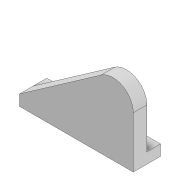
# Autodesk Inventor part: Print_Parts_F1
Saved by Autodesk Inventor 2020 (Build 240168000, 168)
## iProperties
Created: 2020-10-30
Part Number: Print_Parts_F1
Material: Generic
Document SubType Name: Modeling
Designer: magnarecta
Density: 1 g/cm^3
Appearance: Default
Author: magnarecta
Autodesk Inventor part; units mm, degrees
ref_plane "YZ Plane" through (0, 0, 0) normal (1, 0, 0) x (0, 1, 0)
ref_plane "XZ Plane" through (0, 0, 0) normal (0, 1, 0) x (-1, 0, 0)
ref_plane "XY Plane" through (0, 0, 0) normal (0, 0, 1) x (1, 0, 0)
sketch "Sketch1" plane through (0, 0, 0) normal (0, 0, 1) x (1, 0, 0)
  line L0 (0, 0) -> (83.7172, 0)
  line L1 (83.7172, 0) -> (83.7172, 8)
  line L2 (83.7172, 8) -> (0, 8)
  line L3 (0, 8) -> (0, 0)
  line L4 (0, 8) -> (83.7172, 66.6194)
  line L5 (83.7172, 8) -> (83.7172, 66.6194)
  circle A0 centre (68.7172, 37.8047) radius 15
  point P0 (83.7172, 37.8047)
  point P1 (60.1136, 50.092)
  dimension "d0" = 35
  dimension "d1" = 8
  dimension "d12" = 30
  dimension "d13" = 29.8047
  constraints: 12 end point, 2 parallel, 2 tangent, 1 centre point, 1 collinear, 1 horizontal, 1 perpendicular
  measures "d0" angle of L4 L0
  measures "d1" distance of L0.end L1.end
  measures "d12" diameter of A0
  measures "d13" distance from line of A0.centre L2
extrude "Extrusion1" add sketch "Sketch1" along normal blind 10 contours L3 L2 L1 L0 | L4 A0 L5 L2 | A0
sketch "Sketch3" plane through (0, 0, 0) normal (0, 0, -1) x (-1, 0, 0)
  line L0 (-83.7172, 0) -> (-83.7172, 37.8047) projected
  line L1 (0, 0) -> (-83.7172, 0) projected
  line L2 (0, 8) -> (0, 0) projected
  line L3 (-60.1136, 50.092) -> (0, 8) projected
  line L4 (-46.3964, 40.4871) -> (0, 8) projected
  line L5 (-83.7172, 0) -> (0, 0)
  line L6 (0, 0) -> (0, 8)
  line L7 (0, 8) -> (-83.7172, 8)
  line L8 (-83.7172, 8) -> (-83.7172, 0)
  arc A0 (-60.1136, 50.092) -> (-83.7172, 37.8047) centre (-68.7172, 37.8047) ccw projected
  point P0 (-83.7172, 8)
  constraints: 8 end point, 2 parallel, 1 horizontal, 1 perpendicular
extrude "Extrusion3" add sketch "Sketch3" along normal blind 10 contours L0 L7 L2 L1
body "Solid1"
